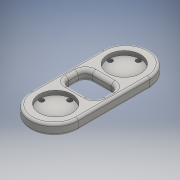
# Autodesk Inventor part: LowerArm
Saved by Autodesk Inventor 2016 (Build 200138000, 138)
## iProperties
Created: 2015-10-06
Part Number: LowerArm
Material: Generic
Document SubType Name: Modeling
Designer: alex
Density: 1 g/cm^3
Appearance: Default
Mass: 56.6565 g
Surface Area: 198.211 cm^2
Volume: 56.6565 cm^3
Author: alex
Autodesk Inventor part; units mm, degrees
ref_plane "YZ Plane" through (0, 0, 0) normal (1, 0, 0) x (0, 1, 0)
ref_plane "XZ Plane" through (0, 0, 0) normal (0, 1, 0) x (-1, 0, 0)
ref_plane "XY Plane" through (0, 0, 0) normal (0, 0, 1) x (1, 0, 0)
sketch "Sketch1" plane through (0, 0, 0) normal (0, 0, 1) x (1, 0, 0)
  line L0 (-20, 50) -> (20, 50)
  line L1 (20, 50) -> (20, -50)
  line L2 (20, -50) -> (-20, -50)
  line L3 (-20, -50) -> (-20, 50)
  point P0 (0, 0)
  dimension "d0" = 50
  dimension "d1" = 50
  dimension "d2" = 20
  dimension "d3" = 20
  constraints: 8 end point, 2 parallel, 1 horizontal, 1 perpendicular
  measures "d0" distance from line of point (0, 0) L0
  measures "d1" distance from line of point (0, 0) L2
  measures "d2" distance from line of point (0, 0) L3
  measures "d3" distance from line of point (0, 0) L1
extrude "Extrusion1" add sketch "Sketch1" along normal blind 9
fillet "Fillet1" radius 20 1 edges at (-20, 50, 4.5)
fillet "Fillet2" radius 20 1 edges at (20, 50, 4.5)
mirror "Mirror1" about plane through (0, 0, 0) normal (0, 1, 0) of "Fillet1", "Fillet2"
fillet "Fillet6" radius 2 8 edges at (14.1422, 44.1422, 0) (-14.1421, 44.1421, 0) (0, 50, 0) (-20, 0, 0) (0.0001, -50, 0) (14.1422, -44.1422, 0) (-14.1421, -44.1421, 0) (20, 0, 0)
fillet "Fillet7" radius 2 8 edges at (14.1422, 44.1422, 9) (0, 50, 9) (-14.1421, 44.1421, 9) (20, 0, 9) (14.1422, -44.1422, 9) (0.0001, -50, 9) (-14.1421, -44.1421, 9) (-20, 0, 9)
sketch "Sketch6" plane through (0, 0, 9) normal (0, 0, 1) x (1, 0, 0)
  circle A0 centre (0, -28.75) radius 13.75
  arc A1 (-18, -30) -> (18, -30) centre (0, -30) ccw projected
  line L0 (18, 30) -> (18, -30) projected
  circle A2 centre (0, -17) radius 2
  circle A3 centre (-11.75, -28.75) radius 2
  circle A4 centre (0, -40.5) radius 2
  circle A5 centre (11.75, -28.75) radius 2
  line L1 (0, 0) -> (-53.5469, 0)
  circle A6 centre (0, 28.75) radius 13.75
  circle A7 centre (0, 17) radius 2
  circle A8 centre (-11.75, 28.75) radius 2
  circle A9 centre (0, 40.5) radius 2
  circle A10 centre (11.75, 28.75) radius 2
  dimension "d41" = 27.5
  dimension "d42" = 5.5
  dimension "d43" = 18
  dimension "d44" = 4
  dimension "d45" = 11.75
  dimension "d46" = 18
  dimension "d49" = 360
  constraints: 10 centre point, 5 symmetric about line, 2 end point, 1 horizontal, 14 other
  measures "d41" diameter of A0
  measures "d43" distance from line of L0 A0.centre
  measures "d44" diameter of A2
  measures "d45" distance of A0.centre A2.centre
  measures "d46" distance from line of L0 A2.centre
extrude "Extrusion6" cut sketch "Sketch6" against normal through all contours A2 | A3 | A4 | A5 | A9 | A8 | A7 | A10
sketch "Sketch8" plane through (0, 0, 9) normal (0, 0, 1) x (1, 0, 0)
  circle A0 centre (0, -28.75) radius 13.75
  line L0 (-18, -30) -> (-18, 30) projected
  arc A1 (-18, -30) -> (18, -30) centre (0, -30) ccw projected
  line L1 (0, 0) -> (-37.1861, 0)
  circle A2 centre (0, 28.75) radius 13.75
  dimension "d62" = 27.5
  dimension "d63" = 18
  dimension "d64" = 1.25
  constraints: 2 centre point, 2 end point, 1 horizontal, 1 symmetric about line, 1 other
  measures "d62" diameter of A0
  measures "d63" distance from line of L0 A0.centre
  measures "d64" distance of A1.centre A0.centre
extrude "Extrusion8" cut sketch "Sketch8" against normal blind 3.5
sketch "Sketch10" plane through (0, 0, 9) normal (0, 0, 1) x (1, 0, 0)
  line L0 (14, -10) -> (-14, -10)
  line L1 (-14, -10) -> (-14, 10)
  line L2 (-14, 10) -> (14, 10)
  line L3 (14, 10) -> (14, -10)
  point P0 (0, 0)
  point P1 (14, 0)
  point P2 (0, -10)
  dimension "d78" = 20
  dimension "d79" = 28
  constraints: 8 end point, 2 midpoint, 2 parallel, 1 horizontal, 1 horizontal alignment, 1 perpendicular, 1 vertical alignment
  measures "d78" distance between parallel lines of L2 L0
  measures "d79" distance between parallel lines of L1 L3
extrude "Extrusion10" cut sketch "Sketch10" against normal through all
fillet "Fillet11" radius 6 4 edges at (14, -10, 4.5) (-14, -10, 4.5) (14, 10, 4.5) (-14, 10, 4.5)
fillet "Fillet12" radius 3 16 edges at (0, -10, 9) (12.2426, -8.2426, 9) (14, 0, 9) (12.2426, 8.2426, 9) (0, 10, 9) (-12.2426, 8.2426, 9) (-14, 0, 9) (-12.2426, -8.2426, 9) (-12.2426, 8.2426, 0) (-14, 0, 0) (-12.2426, -8.2426, 0) (0, -10, 0) (12.2426, -8.2426, 0) (14, 0, 0) (12.2426, 8.2426, 0) (0, 10, 0)
body "Solid1"
